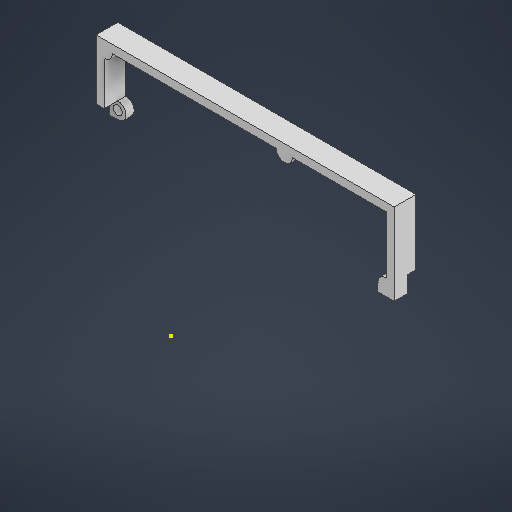
# Autodesk Inventor part: leftwall2
Saved by Autodesk Inventor 2026.2 (Build 302298010, 298A)
## iProperties
Created: 2026-09-07
Part Number: leftwall2
Material: Generic
Document SubType Name: Modeling
Designer: karol
Density: 1 g/cm^3
Appearance: Default
Author: karol
Autodesk Inventor part; units mm, degrees
ref_plane "YZ Plane" through (0, 0, 0) normal (1, 0, 0) x (0, 1, 0)
ref_plane "XZ Plane" through (0, 0, 0) normal (0, 1, 0) x (-1, 0, 0)
ref_plane "XY Plane" through (0, 0, 0) normal (0, 0, 1) x (1, 0, 0)
sketch "Sketch1" plane through (0, 0, 0) normal (0, 0, 1) x (1, 0, 0)
  point P0 (0, 0)
sketch "Sketch2" plane through (0, 0, 0) normal (0, 0, 1) x (1, 0, 0)
  line L0 (-58, -60) -> (-60, -60) projected
  line L1 (-60, -60) -> (-60, -39.5) projected
  line L2 (-60, -39.5) -> (-58, -39.5) projected
  line L3 (-58, -39.5) -> (-58, -60) projected
  line L4 (49.6, 30) -> (51.6, 30) projected
  line L5 (51.6, 30) -> (51.6, 9.5) projected
  line L6 (51.6, 9.5) -> (49.6, 9.5) projected
  line L7 (49.6, 9.5) -> (49.6, 30) projected
  line L8 (-58, 39.5) -> (-60, 39.5) projected
  line L9 (-60, 39.5) -> (-60, 60) projected
  line L10 (-60, 60) -> (-58, 60) projected
  line L11 (-58, 60) -> (-58, 39.5) projected
  line L12 (-21.6, -39.5) -> (-19.6, -39.5) projected
  line L13 (-19.6, -39.5) -> (-19.6, -60) projected
  line L14 (-19.6, -60) -> (-21.6, -60) projected
  line L15 (-21.6, -60) -> (-21.6, -39.5) projected
  line L16 (51.6, -30) -> (49.6, -30) projected
  line L17 (49.6, -30) -> (49.6, -9.5) projected
  line L18 (49.6, -9.5) -> (51.6, -9.5) projected
  line L19 (51.6, -9.5) -> (51.6, -30) projected
  line L20 (-21.6, 60) -> (-19.6, 60) projected
  line L21 (-19.6, 60) -> (-19.6, 39.5) projected
  line L22 (-19.6, 39.5) -> (-21.6, 39.5) projected
  line L23 (-21.6, 39.5) -> (-21.6, 60) projected
  line L24 (90, -35) -> (90, 35) projected
  line L25 (90, 35) -> (49.6, 35) projected
  line L26 (49.6, 35) -> (49.6, 60) projected
  line L27 (49.6, 60) -> (90, 60) projected
  line L28 (90, 60) -> (90, 90) projected
  line L29 (90, 90) -> (-19.6, 90) projected
  line L30 (-19.6, 90) -> (-19.6, 65) projected
  line L31 (-19.6, 65) -> (-60, 65) projected
  line L32 (-60, 65) -> (-60, 90) projected
  line L33 (-60, 90) -> (-90, 90) projected
  line L34 (-90, 90) -> (-90, -90) projected
  line L35 (-90, -90) -> (-60, -90) projected
  line L36 (-60, -90) -> (-60, -65) projected
  line L37 (-60, -65) -> (-19.6, -65) projected
  line L38 (-19.6, -65) -> (-19.6, -90) projected
  line L39 (-19.6, -90) -> (90, -90) projected
  line L40 (90, -90) -> (90, -60) projected
  line L41 (90, -60) -> (49.6, -60) projected
  line L42 (49.6, -60) -> (49.6, -35) projected
  line L43 (49.6, -35) -> (90, -35) projected
  line L44 (86, -32) -> (73.8, -32) projected
  line L45 (73.8, -32) -> (73.8, -7.5) projected
  line L46 (73.8, -7.5) -> (86, -7.5) projected
  line L47 (86, -7.5) -> (86, -32) projected
  line L48 (65.8, -32) -> (53.6, -32) projected
  line L49 (53.6, -32) -> (53.6, -7.5) projected
  line L50 (53.6, -7.5) -> (65.8, -7.5) projected
  line L51 (65.8, -7.5) -> (65.8, -32) projected
  line L52 (86, -86) -> (70.6, -86) projected
  line L53 (70.6, -86) -> (70.6, -69.8) projected
  line L54 (70.6, -69.8) -> (86, -69.8) projected
  line L55 (86, -69.8) -> (86, -86) projected
  line L56 (86, 86) -> (86, 69.8) projected
  line L57 (86, 69.8) -> (70.6, 69.8) projected
  line L58 (70.6, 69.8) -> (70.6, 86) projected
  line L59 (70.6, 86) -> (86, 86) projected
  line L60 (73.8, 32) -> (86, 32) projected
  line L61 (86, 32) -> (86, 7.5) projected
  line L62 (86, 7.5) -> (73.8, 7.5) projected
  line L63 (73.8, 7.5) -> (73.8, 32) projected
  line L64 (65.8, 32) -> (65.8, 7.5) projected
  line L65 (65.8, 7.5) -> (53.6, 7.5) projected
  line L66 (53.6, 7.5) -> (53.6, 32) projected
  line L67 (53.6, 32) -> (65.8, 32) projected
  line L68 (-69.6, -87) -> (-85, -87) projected
  line L69 (-85, -87) -> (-85, -70.8) projected
  line L70 (-85, -70.8) -> (-69.6, -70.8) projected
  line L71 (-69.6, -70.8) -> (-69.6, -87) projected
  line L72 (-56, -62) -> (-56, -37.5) projected
  line L73 (-56, -37.5) -> (-43.8, -37.5) projected
  line L74 (-43.8, -37.5) -> (-43.8, -62) projected
  line L75 (-43.8, -62) -> (-56, -62) projected
  line L76 (-56, 62) -> (-43.8, 62) projected
  line L77 (-43.8, 62) -> (-43.8, 37.5) projected
  line L78 (-43.8, 37.5) -> (-56, 37.5) projected
  line L79 (-56, 37.5) -> (-56, 62) projected
  line L80 (-23.6, 62) -> (-23.6, 37.5) projected
  line L81 (-23.6, 37.5) -> (-35.8, 37.5) projected
  line L82 (-35.8, 37.5) -> (-35.8, 62) projected
  line L83 (-35.8, 62) -> (-23.6, 62) projected
  line L84 (-23.6, -62) -> (-35.8, -62) projected
  line L85 (-35.8, -62) -> (-35.8, -37.5) projected
  line L86 (-35.8, -37.5) -> (-23.6, -37.5) projected
  line L87 (-23.6, -37.5) -> (-23.6, -62) projected
  line L88 (-85, 87) -> (-69.6, 87) projected
  line L89 (-69.6, 87) -> (-69.6, 70.8) projected
  line L90 (-69.6, 70.8) -> (-85, 70.8) projected
  line L91 (-85, 70.8) -> (-85, 87) projected
  line L92 (46.6, 35) -> (49.6, 35) projected
  line L93 (49.6, 35) -> (49.6, 60) projected
  line L94 (49.6, 60) -> (84, 60) projected
  line L95 (84, 63) -> (43.6, 63) projected
  line L96 (46.6, 57) -> (46.6, 35) projected
  line L97 (90, 90) -> (87, 90)
  line L98 (87, 90) -> (87, 63)
  line L99 (87, 63) -> (90, 63)
  line L100 (90, 63) -> (90, 90)
  line L101 (87, 90) -> (-19.6, 90)
  line L102 (-19.6, 90) -> (-19.6, 87)
  line L103 (-19.6, 87) -> (87, 87)
  line L104 (87, 87) -> (87, 90)
  line L105 (-19.6, 90) -> (-16.6, 90)
  line L106 (-16.6, 90) -> (-16.6, 65)
  line L107 (-16.6, 65) -> (-19.6, 65)
  line L108 (-19.6, 65) -> (-19.6, 90)
  line L109 (-19.6, 90) -> (-13.6, 90)
  line L110 (-13.6, 90) -> (-13.6, 84)
  line L111 (-13.6, 84) -> (-19.6, 84)
  line L112 (-19.6, 84) -> (-19.6, 90)
  line L113 (90, 60) -> (84, 60)
  line L114 (84, 60) -> (84, 66)
  line L115 (84, 66) -> (90, 66)
  line L116 (90, 66) -> (90, 60)
  line L117 (-19.6, 65) -> (-16.6, 65)
  line L118 (-16.6, 65) -> (-16.6, 68)
  line L119 (-16.6, 68) -> (-19.6, 68)
  line L120 (-19.6, 68) -> (-19.6, 65)
  line L121 (-19.6, 68) -> (-13.6, 68)
  line L122 (-13.6, 68) -> (-13.6, 62)
  line L123 (-13.6, 62) -> (-19.6, 62)
  line L124 (-19.6, 62) -> (-19.6, 68)
  line L125 (46.6, 90) -> (52.6, 90)
  line L126 (52.6, 90) -> (52.6, 84)
  line L127 (52.6, 84) -> (46.6, 84)
  line L128 (46.6, 84) -> (46.6, 90)
  line L129 (84, 60) -> (84, 63) projected
  circle A0 centre (-63, -65) radius 1.5 projected
  circle A1 centre (-16.6, -87) radius 1.5 projected
  circle A2 centre (49.6, -87) radius 1.5 projected
  circle A3 centre (46.6, -60) radius 1.5 projected
  circle A4 centre (87, -63) radius 1.5 projected
  circle A5 centre (46.6, -32) radius 1.5 projected
  circle A6 centre (46.6, 32) radius 1.5 projected
  circle A7 centre (87, 63) radius 1.5 projected
  circle A8 centre (46.6, 60) radius 1.5 projected
  circle A9 centre (49.6, 87) radius 1.5 projected
  circle A10 centre (-16.6, 87) radius 1.5 projected
  circle A11 centre (-16.6, 65) radius 1.5 projected
  circle A12 centre (-63, 65) radius 1.5 projected
  line L130 (43.6, 63) -> (43.6, 57) projected
  line L131 (43.6, 57) -> (46.6, 57) projected
  point P0 (0, 0)
  point P1 (90, 63)
  point P2 (87, 66)
  point P3 (-16.6, 84)
  point P4 (-13.6, 87)
  point P5 (46.6, 87)
  point P6 (52.6, 87)
  dimension "d0" = 3
  dimension "d1" = 3
  dimension "d2" = 6
  dimension "d3" = 6
  dimension "d4" = 6
  dimension "d5" = 6
  dimension "d6" = 3
  dimension "d7" = 6
  dimension "d8" = 6
  constraints: 64 end point, 16 parallel, 8 horizontal, 8 perpendicular, 4 point on line
  measures "d0" distance of L99.end L98.end
  measures "d1" distance of L106.end L107.end
  measures "d2" distance of L110.end L111.end
  measures "d3" distance of L109.end L110.end
  measures "d4" distance of L114.end L115.end
  measures "d5" distance of L113.end L114.end
  measures "d6" distance of L118.end L117.end
  measures "d7" distance of L126.end L127.end
  measures "d8" distance of L125.end L126.end
extrude "Extrusion1" add sketch "Sketch2" along normal blind 8 contours L114 L115 L98 A7 L99 L28 L27 | L99 A7 L98 L115 L28 | L115 L98 L29 L28 | A7 L98 L99 | L99 L98 A7 | L103 L126 L29 L98 | L126 L127 L128 L103 A9 | L103 A9 L128 L29 L126 | A9 L103 | L103 A9 | L128 L103 L110 L29 | L110 L103 A10 L106 L29 | L106 A10 L103 L30 L29 | L110 L111 L106 A10 L103 | L30 L119 L106 A11 L107 | L107 A11 L106 L121 L122 L123 L124 | A10 L103 L106 | L106 L103 A10 | A10 L106 L103 | L30 L111 L106 L119 | A11 L106 L107 | L107 L106 A11 | L103 A10 L106 L111 L30 | L106 A10 L103
sketch "Sketch3" plane through (0, 0, 0) normal (0, 0, -1) x (-1, 0, 0)
  line L0 (-87, 66) -> (-84, 66) projected
  line L1 (-84, 60) -> (-90, 60) projected
  line L2 (-84, 66) -> (-90, 66)
  line L3 (-90, 66) -> (-90, 60)
  line L4 (-90, 60) -> (-84, 60)
  line L5 (-84, 60) -> (-84, 66)
  point P0 (0, 0)
  constraints: 8 end point, 2 parallel, 1 horizontal, 1 perpendicular
extrude "Extrusion2" cut sketch "Sketch3" against normal blind 3
sketch "Sketch4" plane through (0, 0, 3) normal (0, 0, -1) x (-1, 0, 0)
  line L0 (-87, 66) -> (-84, 66) projected
  line L1 (-90, 60) -> (-90, 90) projected
  line L2 (-84, 66) -> (-90, 60)
  line L3 (-90, 60) -> (-90, 66)
  line L4 (-84, 66) -> (-84, 60) projected
  line L5 (-90, 66) -> (-84, 60)
  circle A0 centre (-87, 63) radius 2
  point P0 (0, 0)
  dimension "d13" = 4
  constraints: 6 end point, 1 centre point, 1 midpoint, 1 perpendicular, 1 vertical
  measures "d13" diameter of A0
extrude "Extrusion3" cut sketch "Sketch4" against normal blind 4 contours A0 L5 L2 | L2 L5 A0 | A0 L2 L5 | L2 A0 L5
sketch "Sketch5" plane through (0, 0, 8) normal (0, 0, 1) x (1, 0, 0)
  line L0 (-13.6, 62) -> (-13.6, 68) projected
  line L1 (-19.6, 62) -> (-13.6, 62) projected
  line L2 (-13.6, 68) -> (-19.6, 68)
  line L3 (-19.6, 68) -> (-19.6, 62)
  line L4 (-19.6, 62) -> (-13.6, 62)
  line L5 (-13.6, 62) -> (-13.6, 68)
  point P0 (0, 0)
  constraints: 8 end point, 2 parallel, 1 horizontal, 1 perpendicular
extrude "Extrusion4" cut sketch "Sketch5" against normal blind 5
sketch "Sketch6" plane through (0, 0, 3) normal (0, 0, 1) x (1, 0, 0)
  line L0 (-13.6, 68) -> (-13.6, 62) projected
  line L1 (-19.6, 62) -> (-19.6, 68) projected
  line L2 (-13.6, 68) -> (-19.6, 62)
  line L3 (-19.6, 62) -> (-19.6, 68)
  line L4 (-19.6, 68) -> (-13.6, 62)
  circle A0 centre (-16.6, 65) radius 1.65
  point P0 (0, 0)
  dimension "d18" = 3.3
  constraints: 6 end point, 1 centre point, 1 collinear, 1 midpoint, 1 perpendicular
  measures "d18" diameter of A0
extrude "Extrusion5" cut sketch "Sketch6" against normal blind 3 contours A0 L4 L2 | L2 L4 A0 | A0 L2 L4 | L2 A0 L4
sketch "Sketch7" plane through (0, 0, 0) normal (0, 0, -1) x (-1, 0, 0)
  point P0 (0, 0)
sketch "Sketch8" plane through (0, 0, 0) normal (0, 0, -1) x (-1, 0, 0)
  line L0 (-46.6, 84) -> (-52.6, 84) projected
  line L1 (-90, 90) -> (19.6, 90) projected
  line L2 (-52.6, 84) -> (-46.6, 84)
  line L3 (-46.6, 84) -> (-46.6, 90)
  line L4 (-46.6, 90) -> (-52.6, 90)
  line L5 (-52.6, 90) -> (-52.6, 84)
  line L6 (-52.6, 84) -> (-46.6, 90)
  line L7 (-46.6, 84) -> (-52.6, 90)
  circle A0 centre (-49.6, 87) radius 2
  line L8 (19.6, 90) -> (13.6, 90)
  line L9 (13.6, 90) -> (13.6, 84)
  line L10 (13.6, 84) -> (19.6, 84)
  line L11 (19.6, 84) -> (19.6, 90)
  line L12 (19.6, 90) -> (13.6, 84) construction
  line L13 (13.6, 90) -> (19.6, 84) construction
  line L14 (13.6, 84) -> (13.6, 87) projected
  circle A1 centre (16.6, 87) radius 2
  point P0 (0, 0)
  dimension "d21" = 6
  dimension "d22" = 4
  dimension "d23" = 6
  dimension "d24" = 6
  dimension "d25" = 4
  constraints: 24 end point, 4 parallel, 3 midpoint, 2 centre point, 2 horizontal, 2 perpendicular, 1 coincident, 1 collinear, 1 point on line
  measures "d21" distance of L4.end L3.end
  measures "d22" diameter of A0
  measures "d23" distance of L10.end L9.end
  measures "d24" distance of L9.end L8.end
  measures "d25" diameter of A1
extrude "Extrusion6" cut sketch "Sketch8" against normal blind 6 contours A0 L6 L7 | L7 L6 A0 | A0 L7 L6 | L6 L7 A0 | A1
fillet "Fillet1" radius 3 4 edges at (-13.6, 62, 1.5) (-13.6, 68, 1.5) (46.6, 84, 4) (52.6, 84, 4)
fillet "Fillet2" radius 3 1 edges at (-13.6, 84, 4)
fillet "Fillet3" radius 3 1 edges at (84, 66, 5.5)
body "Solid1"
